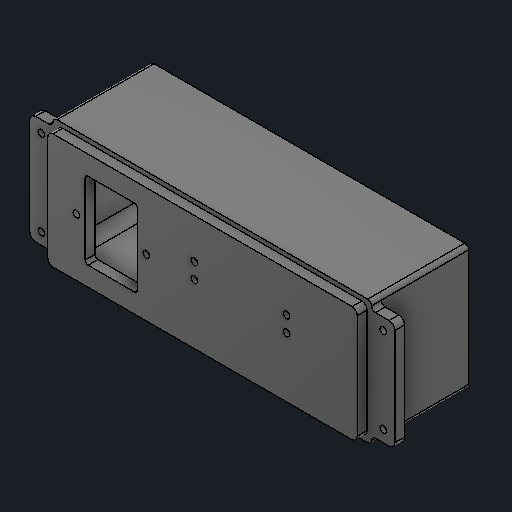
# Autodesk Inventor part: Junction Box Modbay
Saved by Autodesk Inventor 2026.2 (Build 302298000, 298)
## iProperties
Created: 2026-08-18
Part Number: Junction Box Modbay
Material: ABS Plastic
Document SubType Name: Modeling
Designer: JoshuaEah
Density: 1.06 g/cm^3
Appearance: Smooth - Black
Author: JoshuaEah
Autodesk Inventor part; units mm, degrees
ref_plane "YZ Plane" through (0, 0, 0) normal (1, 0, 0) x (0, 1, 0)
ref_plane "XZ Plane" through (0, 0, 0) normal (0, 1, 0) x (-1, 0, 0)
ref_plane "XY Plane" through (0, 0, 0) normal (0, 0, 1) x (1, 0, 0)
sketch "Sketch1" plane through (0, 0, 0) normal (0, 0, 1) x (1, 0, 0)
  line L0 (19.5339, 49.812) -> (46.4579, 49.812)
  line L1 (46.4579, 49.812) -> (46.4579, 10.188)
  line L2 (46.4579, 10.188) -> (19.5339, 10.188)
  line L3 (19.5339, 10.188) -> (19.5339, 49.812)
  line L4 (32.9959, 49.812) -> (32.9959, 10.188)
  line L5 (71.8579, 25.88) -> (71.8579, 44.38)
  line L6 (71.8579, 44.38) -> (127.1079, 44.38)
  line L7 (127.1079, 44.38) -> (127.1079, 25.88)
  line L8 (127.1079, 25.88) -> (71.8579, 25.88)
  line L9 (71.8579, 35.13) -> (127.1079, 35.13)
  line L10 (99.4829, 25.88) -> (99.4829, 44.38)
  line L11 (0, 0) -> (160, 0)
  line L12 (160, 0) -> (160, 60)
  line L13 (160, 60) -> (0, 60)
  line L14 (0, 60) -> (0, 0)
  line L15 (3, 3) -> (157, 3)
  line L16 (157, 3) -> (157, 57)
  line L17 (157, 57) -> (3, 57)
  line L18 (3, 57) -> (3, 3)
  line L19 (0, 58) -> (-14, 58)
  line L20 (-14, 58) -> (-14, 2)
  line L21 (-14, 2) -> (0, 2)
  line L22 (80, 3) -> (80, 57)
  line L23 (160, 58) -> (174, 58)
  line L24 (174, 58) -> (174, 2)
  line L25 (174, 2) -> (160, 2)
  line L26 (-2, 62) -> (162, 62)
  line L27 (162, 62) -> (162, -2)
  line L28 (162, -2) -> (-2, -2)
  line L29 (-2, -2) -> (-2, 62)
  point P0 (15, 30)
  point P1 (32.9959, 30)
  point P2 (50.9918, 30)
  point P3 (19.5339, 30)
  point P4 (75.7329, 31.13)
  point P5 (123.2329, 31.13)
  point P6 (75.7329, 39.13)
  point P7 (123.2329, 39.13)
  point P8 (99.4829, 35.13)
  point P9 (0, 30)
  point P10 (-8, 52)
  point P11 (-8, 8)
  point P12 (168, 52)
  point P13 (168, 8)
  dimension "d0" = 26.924
  dimension "d1" = 39.624
  dimension "d2" = 35.9918
  dimension "d3" = 18.5
  dimension "d4" = 55.25
  dimension "d6" = 8
  dimension "d7" = 3.875
  dimension "d21" = 160
  dimension "d24" = 60
  dimension "d27" = 25.4
  dimension "d28" = 15
  dimension "d33" = 8
  dimension "d34" = 8
  dimension "d35" = 8
  dimension "d36" = 6
  dimension "d37" = 6
  dimension "d38" = 6
  dimension "d50" = 3
  dimension "d51" = 4
  constraints: 60 end point, 12 midpoint, 10 parallel, 10 symmetric about line, 8 perpendicular, 2 horizontal, 2 horizontal alignment, 2 point on line, 1 coincident, 1 vertical alignment, 6 other
  measures "d0" distance of L1.end L2.end
  measures "d1" distance of L0.end L1.end
  measures "d2" diameter of point (15, 30) L4
  measures "d3" distance of L6.end L7.end
  measures "d4" distance of L7.end L5.start
  measures "d6" diameter of point (75.733, 31.13) L9
  measures "d7" distance from line of L5 point (75.733, 31.13)
  measures "d21" distance of L12.end L13.end
  measures "d24" distance of L13.end L11.start
  measures "d27" distance between parallel lines of L1 L5
  measures "d28" distance from line of L14 point (15, 30)
  measures "d33" distance from line of L14 point (-8, 52)
  measures "d34" distance from line of L13 point (-8, 52)
  measures "d35" distance from line of L11 point (-8, 8)
  measures "d36" distance from line of point (-8, 8) L21
  measures "d37" distance from line of L20 point (-8, 8)
  measures "d38" distance from line of point (-8, 52) L19
  measures "d50" distance between parallel lines of L13 L17
  measures "d51" distance between parallel lines of L26 L19
extrude "Extrusion1" add sketch "Sketch1" along normal blind 5 contours L8 L22 L15 L18 L17 L6 L5 | L5 L9 L22 L8 | L5 L6 L22 L9 | L22 L9 L10 L8 | L8 L7 L6 L22 L17 L16 L15 | L22 L6 L10 L9 | L10 L9 L7 L8 | L10 L6 L7 L9 | L14 L13 L12 L11
fillet "Fillet1" radius 1.524 4 edges at (19.5339, 49.812, 2.5) (46.4579, 49.812, 2.5) (46.4579, 10.188, 2.5) (19.5339, 10.188, 2.5)
hole "Hole1" at (15, 30, 0) at (50.9918, 30, 0) at (75.7329, 31.13, 0) at (123.2329, 31.13, 0) at (75.7329, 39.13, 0) at (123.2329, 39.13, 0) direction (0, 0, 1) diameter 3.4036 end through all start extended yes clearance for "Socket Head Cap Screw" size "M3" standard "Ansi Metric M Profile"
extrude "Extrusion2" add sketch "Sketch1" against normal blind 50 contours L14 L13 L12 L11 | L11 L12 L25 L27 L28 L29 L21 L14 | L21 L29 L19 L14 | L12 L23 L27 L25 | L19 L29 L26 L27 L23 L12 L13 L14
extrude "Extrusion3" add sketch "Sketch1" against normal blind 5 contours L21 L29 L19 L14 | L12 L23 L27 L25 | L21 L20 L19 L29 | L27 L23 L24 L25
fillet "Fillet2" radius 3 4 edges at (0, 60, 2.5) (160, 60, 2.5) (0, 0, 2.5) (160, 0, 2.5)
fillet "Fillet3" radius 3 4 edges at (-14, 58, -2.5) (-14, 2, -2.5) (174, 58, -2.5) (174, 2, -2.5)
fillet "Fillet3" radius 2 8 edges at (-2, 62, -25) (162, 62, -25) (162, -2, -25) (-2, -2, -25) (-2, 2, -2.5) (-2, 58, -2.5) (162, 58, -2.5) (162, 2, -2.5)
hole "Hole2" at (-8, 52, 0) at (-8, 8, 0) at (168, 52, 0) at (168, 8, 0) direction (0, 0, -1) diameter 3.4036 end through all start extended yes clearance for "Flat Head Machine Screw" size "M3" standard "Ansi Metric M Profile"
thicken "Thicken1" operation add thickness 0.3 both sides no extend neighbours yes toward (0, -1, 0) faces at (105.6667, 60, 1.6667) (0.0335, 57.4471, 1.6667) (0, 21, 3.3333) (1.904, 0.2074, 1.6667) (54.3333, 0, 1.6667) (160, 39, 3.3333) (158.096, 59.7926, 1.6667)
fillet "Fillet4" radius 3 4 edges at (157, 57, -25) (3, 57, -25) (3, 3, -25) (157, 3, -25)
thicken "Thicken2" operation add thickness 2 both sides no extend neighbours yes toward (0, 1, 0) faces at (55.3333, 57, -16.6667) (154.8843, 56.8667, -16.6667) (157, 38, -16.6667) (154.8843, 3.1333, -16.6667) (104.6667, 3, -16.6667) (3.0084, 5.7758, -16.6667) (3, 22, -16.6667) (3.4019, 55.5, -16.6667)
equation "\"d34\" = d33"
equation "\"d35\" = d34"
equation "\"d37\" = d36"
body "Solid1"
